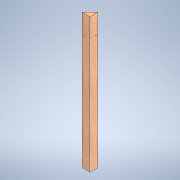
# Autodesk Inventor part: coluna
Saved by Autodesk Inventor 2022 (Build 260153000, 153)
## iProperties
Created: 2022-02-16
Part Number: coluna
Material: Madeira (Bétula)
Document SubType Name: Modeling
Designer: mathe
Density: 0.55 g/cm^3
Appearance: Bétula - Natural polido
Author: mathe
Autodesk Inventor part; units mm, degrees
ref_plane "YZ Plane" through (0, 0, 0) normal (1, 0, 0) x (0, 1, 0)
ref_plane "XZ Plane" through (0, 0, 0) normal (0, 1, 0) x (-1, 0, 0)
ref_plane "XY Plane" through (0, 0, 0) normal (0, 0, 1) x (1, 0, 0)
sketch "Esboço1" plane through (0, 0, 0) normal (0, 1, 0) x (-1, 0, 0)
  line L0 (0, 0) -> (40, 0)
  line L1 (0, -40) -> (0, 0)
  line L2 (0, -40) -> (40, 0)
  constraints: 6 end point, 1 horizontal
extrude "Extrusão1" add sketch "Esboço1" along normal blind 700
sketch "Esboço2" plane through (-40, 0, 0) normal (-0.7071068, 0, -0.7071068) x (-0.7071068, 0, 0.7071068)
  line L0 (0, 700) -> (-28.2843, 700) projected
  line L1 (-28.2843, 700) -> (-28.2843, 600)
  line L2 (-28.2843, 0) -> (-28.2843, 700) projected
  line L3 (-28.2843, 600) -> (-6.7843, 600)
  line L4 (-6.7843, 600) -> (-28.2843, 600)
  line L5 (-28.2843, 600) -> (-49.7843, 600)
  dimension "d4" = 100
  dimension "d5" = 21.5
  dimension "d6" = 21.5
  constraints: 8 end point, 2 coincident, 2 horizontal, 1 collinear, 1 point on line
  measures "d4" distance of L0.end L1.end
  measures "d5" distance of L1.end L3.end
  measures "d6" distance of L1.end L5.end
hole "Furo1" at (-35.2028, 600, -4.7972) at (-4.7972, 600, -35.2028) direction (0.7071068, 0, 0.7071068) diameter 3 end through all
